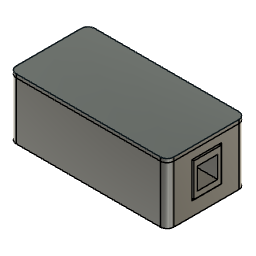
enclosure (Autodesk Fusion 360 design; units mm, degrees)
Autodesk Fusion 360 part; units mm, degrees
sketch "Sketch1" plane through (0, 0, 0) normal (0, 0, 1) x (1, 0, 0) in component "DSMR reader"
  line L0 (-32.9574, 13.5458) -> (33.0426, 13.5458)
  line L1 (33.0426, 13.5458) -> (33.0426, -13.4542)
  line L2 (33.0426, -13.4542) -> (-32.9574, -13.4542)
  line L3 (-32.9574, -13.4542) -> (-32.9574, 13.5458)
  circle A0 centre (-30.456, 10.9724) radius 1.6
  line L4 (0.0426, 13.5458) -> (0.0426, -13.4542) construction
  line L5 (-32.9574, 0.0458) -> (33.0426, 0.0458) construction
  circle A1 centre (30.5413, 10.9724) radius 1.6
  circle A2 centre (30.5413, -10.8808) radius 1.6
  circle A3 centre (-30.456, -10.8808) radius 1.6
  line L6 (22.5426, 6.2479) -> (35.5426, 6.2479)
  line L7 (35.5426, 6.2479) -> (35.5426, -6.0334)
  line L8 (35.5426, -6.0334) -> (22.5426, -6.0334)
  line L9 (22.5426, -6.0334) -> (22.5426, 6.2479)
  circle A4 centre (29.5, 6.1421) radius 1.2402
  circle A5 centre (29.5, -5.9879) radius 1.2402
  dimension "d1" = 66
  dimension "d2" = 27
  dimension "d3" = 3.2
  dimension "d6" = 2.5
  constraint horizontal L0
  constraint vertical L1
  constraint horizontal L2
  constraint vertical L3
  constraint midpoint L0 L4.start
  constraint midpoint L2 L4.end
  constraint midpoint L3 L5.start
  constraint midpoint L1 L5.end
  constraint symmetric A0 L4 A1
  constraint symmetric L5 A1 A2
  constraint symmetric A0 L5 A3
  constraint horizontal L6
  constraint vertical L7
  constraint horizontal L8
  constraint vertical L9
  measures "d1" distance of L1.end L2.end
  measures "d2" distance of L0.start L2.end
  measures "d3" diameter of A0
  measures "d6" distance of L1 L7
extrude "Extrude1" add sketch "Sketch1" against normal blind 1.6 contours L0 L1 L2 L3 L6 L8 L9 A4 A5 | L1 L6 L8 L9 A4 A5 makes body 1 in component "DSMR reader"
extrude "Extrude2" add sketch "Sketch1" along normal blind 15 contours L1 L6 L7 L8 | L1 L6 L8 L9 A4 A5 bodies 1 in component "DSMR reader"
extrude "Extrude3" add sketch "Sketch1" along normal blind 15 separate body contours L6 A4 | L6 A4 | L8 A5 | L8 A5 makes body 2 at (30.734, -5.8644, 10) makes body 3 at (30.734, 6.0187, 5) in component "DSMR reader"
sketch "Sketch1 (2)" plane through (0, 0, 0) normal (0, 0, 1) x (1, 0, 0) in component "Box"
  line L0 (-33.9574, 16) -> (33.5426, 16)
  line L1 (33.5426, 16) -> (33.5426, -16)
  line L2 (33.5426, -16) -> (-33.9574, -16)
  line L3 (-33.9574, -16) -> (-33.9574, 16)
  line L4 (22.5426, 6.2479) -> (28.2643, 6.2479)
  arc A0 (30.7356, 6.2479) -> (28.2643, 6.2479) centre (29.5, 6.1421) ccw
  line L5 (30.7356, 6.2479) -> (33.0426, 6.2479)
  line L6 (33.0426, 6.2479) -> (33.0426, 13.5458)
  line L7 (33.0426, 13.5458) -> (-32.9574, 13.5458)
  line L8 (-32.9574, 13.5458) -> (-32.9574, -13.4542)
  line L9 (-32.9574, -13.4542) -> (33.0426, -13.4542)
  line L10 (33.0426, -13.4542) -> (33.0426, -6.0334)
  line L11 (33.0426, -6.0334) -> (30.7393, -6.0334)
  arc A1 (28.2606, -6.0334) -> (30.7393, -6.0334) centre (29.5, -5.9879) ccw
  line L12 (28.2606, -6.0334) -> (22.5426, -6.0334)
  line L13 (22.5426, -6.0334) -> (22.5426, 6.2479)
  circle A2 centre (-30.456, 10.9724) radius 1.6
  circle A3 centre (-30.456, -10.8808) radius 1.6
  circle A4 centre (30.5413, -10.8808) radius 1.6
  circle A5 centre (30.5413, 10.9724) radius 1.6
  line L14 (35.5426, -6.0334) -> (35.5426, 6.2479)
  line L15 (35.5426, 6.2479) -> (30.7356, 6.2479)
  line L16 (30.7393, -6.0334) -> (35.5426, -6.0334)
  circle A6 centre (30.5413, 10.9724) radius 1.6
  circle A7 centre (30.5413, -10.8808) radius 1.6
  line L17 (-32.9574, 13.5458) -> (33.0426, 13.5458)
  line L18 (-32.9574, -13.4542) -> (-32.9574, 13.5458)
  line L19 (33.0426, -13.4542) -> (-32.9574, -13.4542)
  line L20 (-33.9574, 0) -> (0, 0) construction
  line L21 (35.1426, -17.6) -> (-35.5574, -17.6)
  line L22 (-35.5574, -17.6) -> (-35.5574, 17.6)
  line L23 (-35.5574, 17.6) -> (35.1426, 17.6)
  line L24 (35.1426, 17.6) -> (35.1426, -17.6)
  circle A8 centre (-30.456, 10.9724) radius 2.5
  circle A9 centre (-30.456, 10.9724) radius 0.9
  line L25 (0.0426, 13.5458) -> (0.0426, -1.8412) construction
  circle A10 centre (30.5413, 10.9724) radius 0.9
  circle A11 centre (30.5413, 10.9724) radius 2.5
  circle A12 centre (30.5413, -10.9724) radius 2.5
  circle A13 centre (30.5413, -10.9724) radius 0.9
  circle A14 centre (-30.456, -10.9724) radius 0.9
  circle A15 centre (-30.456, -10.9724) radius 2.5
  dimension "d13" = 0.5
  dimension "d14" = 1
  dimension "d15" = -1.6
  dimension "d16" = 32
  dimension "d27" = 5
  dimension "d28" = -0.7
  constraint horizontal L0
  constraint vertical L1
  constraint horizontal L2
  constraint vertical L3
  constraint midpoint L3 L20.start
  constraint coincident L20.end origin
  constraint horizontal L20
  constraint concentric A2 A8
  constraint midpoint L17 L25.start
  constraint perpendicular L7 L25
  constraint symmetric A8 L25 A11
  constraint symmetric A9 L25 A10
  constraint symmetric L20 A8 A15
  constraint symmetric L20 A9 A14
  constraint symmetric L20 A10 A13
  constraint symmetric L20 A11 A12
  measures "d13" distance of L1 L10
  measures "d14" distance of L3 L8
  measures "d16" distance of L0 L2
  measures "d27" diameter of A8
combine "Combine1" operation add target body 1 tool bodies 2 3 in component "DSMR reader"
extrude "Extrude1'" add sketch "Sketch1 (2)" against normal blind 5 separate body contours L0 L1 L2 L3 L15 L16 L21 L22 L23 L24 | L1 L15 L16 L24 makes body 4 in component "Box"
extrude "Extrude2'" add sketch "Sketch1 (2)" along normal blind 19 contours L0 L1 L2 L3 L15 L16 L21 L22 L23 L24 bodies 4 in component "Box"
fillet "Fillet1" radius 3 4 edges at (-33.9574, 16, 7) (-33.9574, -16, 7) (33.5426, 16, 7) (33.5426, -16, 7) on bodies 4 in component "Box"
fillet "Fillet2" radius 3 4 edges at (35.1426, 17.6, 7) (-35.5574, 17.6, 7) (-35.5574, -17.6, 7) (35.1426, -17.6, 7) on bodies 4 in component "Box"
sketch "Sketch2" plane through (0, 0, -5) normal (0, 0, -1) x (1, 0, 0) in component "Box"
  arc A0 (35.1426, 14.6) -> (32.1426, 17.6) centre (32.1426, 14.6) ccw
  line L0 (32.1426, 17.6) -> (-32.5574, 17.6)
  arc A1 (-32.5574, 17.6) -> (-35.5574, 14.6) centre (-32.5574, 14.6) ccw
  line L1 (-35.5574, 14.6) -> (-35.5574, -14.6)
  arc A2 (-35.5574, -14.6) -> (-32.5574, -17.6) centre (-32.5574, -14.6) ccw
  line L2 (-32.5574, -17.6) -> (32.1426, -17.6)
  arc A3 (32.1426, -17.6) -> (35.1426, -14.6) centre (32.1426, -14.6) ccw
  line L3 (35.1426, -14.6) -> (35.1426, 14.6)
  line L4 (-30.9574, 16) -> (30.5426, 16)
  arc A4 (33.5426, 13) -> (30.5426, 16) centre (30.5426, 13) ccw
  line L5 (33.5426, 13) -> (33.5426, -13)
  arc A5 (30.5426, -16) -> (33.5426, -13) centre (30.5426, -13) ccw
  line L6 (30.5426, -16) -> (-30.9574, -16)
  arc A6 (-33.9574, -13) -> (-30.9574, -16) centre (-30.9574, -13) ccw
  line L7 (-33.9574, -13) -> (-33.9574, 13)
  arc A7 (-30.9574, 16) -> (-33.9574, 13) centre (-30.9574, 13) ccw
  arc A8 (32.1426, -17.6) -> (35.1426, -14.6) centre (32.1426, -14.6) ccw
  line L8 (35.1426, -17.6) -> (35.1426, 17.6)
  arc A9 (35.1426, 14.6) -> (32.1426, 17.6) centre (32.1426, 14.6) ccw
  line L9 (35.1426, 17.6) -> (-35.5574, 17.6)
  arc A10 (-32.5574, 17.6) -> (-35.5574, 14.6) centre (-32.5574, 14.6) ccw
  line L10 (-35.5574, 17.6) -> (-35.5574, -17.6)
  arc A11 (-35.5574, -14.6) -> (-32.5574, -17.6) centre (-32.5574, -14.6) ccw
  line L11 (-35.5574, -17.6) -> (35.1426, -17.6)
extrude "Extrude3'" add sketch "Sketch2" along normal blind 1.6 contours A0 L0 A1 L1 A2 L2 A3 L3 A8 L8 A9 L9 A10 L10 A11 L11 | L4 A4 L5 A5 L6 A6 L7 A7 bodies 4 in component "Box"
extrude "Extrude4" add sketch "Sketch1 (2)" against normal up to surface (3.4 mm away) from surface at -1.6 contours A11 | L9 L19 A12 | L9 L19 A15 | A2 | A3 | A4 A7 | A5 A6 | A8 picked at (30.5812, -13.1283) picked at (-30.4959, -13.1283) bodies 4 in component "Box"
extrude "Extrude1''" add sketch "Sketch2" against normal blind 1.6 from surface at -24 separate body contours A0 L0 A1 L1 A2 L2 A3 L3 A8 L8 A9 L9 A10 L10 A11 L11 | L4 A4 L5 A5 L6 A6 L7 A7 makes body 5 in component "Lid"
sketch "Sketch3" plane through (0, 0, 19) normal (0, 0, -1) x (1, 0, 0) in component "Box"
  line L0 (-32.5574, -17.6) -> (32.1426, -17.6)
  arc A0 (32.1426, -17.6) -> (35.1426, -14.6) centre (32.1426, -14.6) ccw
  line L1 (35.1426, -14.6) -> (35.1426, 14.6)
  arc A1 (35.1426, 14.6) -> (32.1426, 17.6) centre (32.1426, 14.6) ccw
  line L2 (32.1426, 17.6) -> (-32.5574, 17.6)
  arc A2 (-32.5574, 17.6) -> (-35.5574, 14.6) centre (-32.5574, 14.6) ccw
  line L3 (-35.5574, 14.6) -> (-35.5574, -14.6)
  arc A3 (-35.5574, -14.6) -> (-32.5574, -17.6) centre (-32.5574, -14.6) ccw
extrude "Extrude2''" add sketch "Sketch2" along normal blind 2 from surface at -24 contours L4 A4 L5 A5 L6 A6 L7 A7 bodies 5 in component "Lid"
sketch "Sketch1 (3)" plane through (0, 0, 17) normal (0, 0, -1) x (1, 0, 0) in component "Lid"
  line L0 (30.5426, 16) -> (-30.9574, 16)
  arc A0 (-30.9574, 16) -> (-33.9574, 13) centre (-30.9574, 13) ccw
  line L1 (-33.9574, 13) -> (-33.9574, -13)
  arc A1 (-33.9574, -13) -> (-30.9574, -16) centre (-30.9574, -13) ccw
  line L2 (-30.9574, -16) -> (30.5426, -16)
  arc A2 (30.5426, -16) -> (33.5426, -13) centre (30.5426, -13) ccw
  line L3 (33.5426, -13) -> (33.5426, 13)
  arc A3 (33.5426, 13) -> (30.5426, 16) centre (30.5426, 13) ccw
sketch "Sketch2 (2)" plane through (0, 0, 17) normal (0, 0, -1) x (1, 0, 0) in component "Lid"
  line L0 (-30.9574, 16) -> (30.5426, 16)
  arc A0 (-30.9574, 16) -> (-33.9574, 13) centre (-30.9574, 13) ccw
  line L1 (-33.9574, -13) -> (-33.9574, 13)
  arc A1 (-33.9574, -13) -> (-30.9574, -16) centre (-30.9574, -13) ccw
  line L2 (30.5426, -16) -> (-30.9574, -16)
  arc A2 (30.5426, -16) -> (33.5426, -13) centre (30.5426, -13) ccw
  line L3 (33.5426, 13) -> (33.5426, -13)
  arc A3 (33.5426, 13) -> (30.5426, 16) centre (30.5426, 13) ccw
  arc A4 (32.3426, 13) -> (30.5426, 14.8) centre (30.5426, 13) ccw
  line L4 (-30.9574, 14.8) -> (30.5426, 14.8)
  arc A5 (-30.9574, 14.8) -> (-32.7574, 13) centre (-30.9574, 13) ccw
  line L5 (-32.7574, -13) -> (-32.7574, 13)
  arc A6 (-32.7574, -13) -> (-30.9574, -14.8) centre (-30.9574, -13) ccw
  line L6 (30.5426, -14.8) -> (-30.9574, -14.8)
  arc A7 (30.5426, -14.8) -> (32.3426, -13) centre (30.5426, -13) ccw
  line L7 (32.3426, 13) -> (32.3426, -13)
  dimension "d38" = -1.2
extrude "Extrude4'" cut sketch "Sketch2 (2)" against normal blind 2 contours A4 L4 A5 L5 A6 L6 A7 L7 bodies 1 in component "DSMR reader"
extrude "Extrude3''" cut sketch "Sketch2 (2)" against normal blind 2 contours A4 L4 A5 L5 A6 L6 A7 L7 bodies 5 in component "Lid"
move_face "OffsetFaces1" offset -0.5 2 faces at (34.6093, 6.2479, 6.3333) (34.076, -6.0334, 6.3333) on bodies 4 in component "Box"
sketch "Sketch1 (4)" plane through (0, 6.7479, 0) normal (0, -1, 0) x (1, 0, 0)
  line L0 (33.5426, 0) -> (35.1426, 0)
  line L1 (35.1426, 0) -> (35.1426, 19)
  line L2 (35.1426, 19) -> (33.5426, 19)
  line L3 (33.5426, 19) -> (33.5426, 0)
  line L4 (35.1426, 19) -> (33.5426, 19)
  line L5 (33.5426, 19) -> (33.5426, 15.5)
  line L6 (33.5426, 15.5) -> (35.1426, 15.5)
  line L7 (35.1426, 15.5) -> (35.1426, 19)
  point P0 (35.5426, 15)
  dimension "d45" = 0.5
  constraint horizontal L4
  constraint vertical L5
  constraint horizontal L6
  constraint vertical L7
  constraint coincident L3 L5.end
  constraint coincident L1.end L2.start
  measures "d45" distance of P0 L6
extrude "Extrude5" add sketch "Sketch1 (4)" along normal up to surface (13.2813 mm away) contours L1 L2 L3 L4 L5 L6 L7 bodies 4 in component "Box"
move_face "OffsetFaces2" offset -0.5 1 faces at (34.6093, -2.1063, 0) on bodies 4 in component "Box"
ref_plane "WorkPlane1" through (-0.2074, 0, 18) normal (1, 0, 0) x (0, -1, 0)
sketch "Sketch2 (3)" plane through (-33.9574, 0, 0) normal (-1, 0, 0) x (0, -1, 0)
  line L0 (13, 19) -> (-13, 19)
  line L1 (-13, 19) -> (-13, 17)
  line L2 (-13, 17) -> (13, 17)
  line L3 (13, 17) -> (13, 19)
  line L4 (-6, 18.5) -> (6, 18.5)
  line L5 (6, 18.5) -> (6, 17)
  line L6 (6, 17) -> (-6, 17)
  line L7 (-6, 17) -> (-6, 18.5)
  line L8 (0, 19) -> (0, 18.5) construction
  line L9 (13, 17) -> (-13, 17) construction
  dimension "d49" = 1.5
  dimension "d50" = 12
  constraint horizontal L4
  constraint vertical L5
  constraint horizontal L6
  constraint vertical L7
  constraint midpoint L0 L8.start
  constraint midpoint L4 L8.end
  constraint vertical L8
  constraint collinear L6 L9
  measures "d49" distance of L4.end L5.end
  measures "d50" distance of L4.start L4.end
extrude "Extrude4''" add sketch "Sketch2 (3)" along normal blind 1 draft -45 contours L2 L4 L5 L6 L7 bodies 5 in component "Lid"
mirror "Mirror1" about plane through (-0.2074, 0, 18) normal (1, 0, 0) of "Extrude4''" in component "Lid"
combine "Combine1'" operation cut target body 4 tool bodies 5 keep tools in component "Box"
move_face "OffsetFaces3" offset -0.1 8 faces at (33.7926, 1.75, 17.25) (33.7926, 5.75, 17.75) (33.7926, 1.75, 18.25) (33.7926, -5.75, 17.75) (-34.2074, -5.75, 17.75) (-34.2074, 1.75, 17.25) (-34.2074, 1.75, 18.25) (-34.2074, 5.75, 17.75) on bodies 4 in component "Box"
move_face "OffsetFaces1'" offset -0.1 8 faces at (-10.4574, -16, 18.3333) (-33.7924, -13.9812, 17.6667) (-33.9574, 10.6667, 18.1667) (-32.3321, 15.6665, 17.6667) (10.0426, 16, 18.3333) (32.2828, 15.4437, 17.6667) (33.5426, 10.6667, 18.1667) (31.9173, -15.6665, 17.6667) on bodies 5 in component "Lid"
sketch "Sketch3 (2)" plane through (0, 0, -6.6) normal (0, 0, -1) x (1, 0, 0)
  arc A0 (-35.5574, -14.6) -> (-32.5574, -17.6) centre (-32.5574, -14.6) ccw
  line L0 (-32.5574, -17.6) -> (32.1426, -17.6)
  arc A1 (32.1426, -17.6) -> (35.1426, -14.6) centre (32.1426, -14.6) ccw
  line L1 (35.1426, -14.6) -> (35.1426, 14.6)
  arc A2 (35.1426, 14.6) -> (32.1426, 17.6) centre (32.1426, 14.6) ccw
  line L2 (32.1426, 17.6) -> (-32.5574, 17.6)
  arc A3 (-32.5574, 17.6) -> (-35.5574, 14.6) centre (-32.5574, 14.6) ccw
  line L3 (-35.5574, 14.6) -> (-35.5574, -14.6)
  line L4 (0, 0) -> (35.1426, 0) construction
  line L5 (-35.5574, 0) -> (0, 0) construction
  line L6 (-17.7787, 0) -> (-17.7787, 7.2149) construction
  line L7 (17.5713, 0) -> (17.5713, 6.7243) construction
  line L8 (14.5713, 1.6) -> (20.5713, 1.6)
  line L9 (20.5713, -1.6) -> (14.5713, -1.6)
  line L10 (14.5713, 0) -> (17.5713, 0) construction
  line L11 (17.5713, 1.6) -> (17.5713, 0) construction
  arc A4 (14.5713, 1.6) -> (14.5713, -1.6) centre (14.5713, 0) ccw
  arc A5 (20.5713, -1.6) -> (20.5713, 1.6) centre (20.5713, 0) ccw
  line L12 (-19.3787, -3) -> (-16.1787, -3)
  line L13 (-16.1787, -3) -> (-16.1787, 3)
  line L14 (-16.1787, 3) -> (-19.3787, 3)
  line L15 (-19.3787, 3) -> (-19.3787, -3)
  line L16 (-19.3787, 0) -> (-17.7787, 0) construction
  line L17 (-17.7787, 3) -> (-17.7787, 0) construction
  arc A6 (-19.3787, -3) -> (-16.1787, -3) centre (-17.7787, -3) ccw
  arc A7 (-16.1787, 3) -> (-19.3787, 3) centre (-17.7787, 3) ccw
  dimension "d57" = 3.2
  dimension "d58" = 6
  dimension "d59" = 1.6
  dimension "d60" = 3.2
  dimension "d61" = 6
  dimension "d62" = 1.6
  dimension "d63" = 3.2
  dimension "d64" = 6
  constraint coincident L4.start L5.end
  constraint midpoint L1 L4.end
  constraint midpoint L3 L5.start
  constraint midpoint L5 L6.start
  constraint perpendicular L5 L6
  constraint midpoint L4 L7.start
  constraint perpendicular L4 L7
  constraint horizontal L8
  constraint horizontal L9
  constraint midpoint L8 L11.start
  constraint vertical L11
  constraint horizontal L10
  constraint tangent L9 A4
  constraint tangent L9 A5
  constraint horizontal L12
  constraint vertical L13
  constraint horizontal L14
  constraint vertical L15
  constraint midpoint L15 L16.start
  constraint midpoint L14 L17.start
  constraint vertical L17
  constraint horizontal L16
  constraint tangent L13 A7
  constraint tangent L13 A6
  measures "d57" distance of L8.start L9.end
  measures "d58" distance of L8.start L8.end
  measures "d59" distance of L8 L10.start
  measures "d60" distance of L8 L9
  measures "d61" distance of L10.start A5.centre
  measures "d62" radius of A5
  measures "d63" distance of L13.end L14.end
  measures "d64" distance of L12.start L14.end
extrude "Extrude6" cut sketch "Sketch3 (2)" against normal up to surface (1.6 mm away) contours L8 L9 A4 A5 | L12 L13 L14 L15 | L12 A6 | L14 A7 bodies 4 in component "Box"
chamfer "Chamfer1" distance 0.8 angle 45 4 edges at (-16.1787, 0, -5) (-17.7787, -4.6, -5) (-19.3787, 0, -5) (-17.7787, 4.6, -5) on bodies 4 in component "Box"
chamfer "Chamfer1" distance 0.8 angle 45 4 edges at (17.5713, 1.6, -5) (22.1713, 0, -5) (17.5713, -1.6, -5) (12.9713, 0, -5) on bodies 4 in component "Box"
sketch "Sketch4" plane through (35.5426, 0, 0) normal (1, 0, 0) x (0, 1, 0)
  line L0 (-6.0334, 0) -> (6.2479, 0)
  line L1 (6.2479, 0) -> (6.2479, 15)
  line L2 (6.2479, 15) -> (-6.0334, 15)
  line L3 (-6.0334, 15) -> (-6.0334, 0)
  line L4 (-4.4334, 13.2) -> (4.6479, 13.2)
  line L5 (4.6479, 13.2) -> (4.6479, 2.5)
  line L6 (4.6479, 2.5) -> (-4.4334, 2.5)
  line L7 (-4.4334, 2.5) -> (-4.4334, 13.2)
  dimension "d69" = 1.8
  dimension "d70" = 1.6
  dimension "d71" = 1.6
  dimension "d72" = 2.5
  constraint horizontal L4
  constraint vertical L5
  constraint horizontal L6
  constraint vertical L7
  measures "d69" distance of L2 L4
  measures "d70" distance of L3 L7
  measures "d71" distance of L1 L5
  measures "d72" distance of L0 L6
extrude "Extrude5'" cut sketch "Sketch4" against normal blind 11 contours L4 L5 L6 L7 bodies 1 in component "DSMR reader"
extrude "Extrude6'" add 1 faces at (31.876, -1.4063, 13.2) along direction (0, 0, -1) blind 1 on bodies 1 bodies 1 in component "DSMR reader"
sketch "Sketch5" plane through (0, 0, 20.6) normal (0, 0, 1) x (-1, 0, 0)
  line L0 (-32.1426, -17.6) -> (32.5574, -17.6)
  arc A0 (32.5574, -17.6) -> (35.5574, -14.6) centre (32.5574, -14.6) ccw
  line L1 (35.5574, -14.6) -> (35.5574, 14.6)
  arc A1 (35.5574, 14.6) -> (32.5574, 17.6) centre (32.5574, 14.6) ccw
  line L2 (32.5574, 17.6) -> (-32.1426, 17.6)
  arc A2 (-32.1426, 17.6) -> (-35.1426, 14.6) centre (-32.1426, 14.6) ccw
  line L3 (-35.1426, 14.6) -> (-35.1426, -14.6)
  arc A3 (-35.1426, -14.6) -> (-32.1426, -17.6) centre (-32.1426, -14.6) ccw
component "DSMR reader" placed x (1, 0, 0) y (0, 1, 0) z (0, 0, 1) at (0, 0, 0)
component "Box" placed x (1, 0, 0) y (0, 1, 0) z (0, 0, 1) at (0, 0, 0)
component "Lid" placed x (1, 0, 0) y (0, 1, 0) z (0, 0, 1) at (0, 0, 0) in component "Box"
